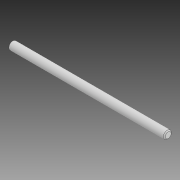
# Autodesk Inventor part: M8x160mm Threaded Rod
Saved by Autodesk Inventor 2020 (Build 240168000, 168)
## iProperties
Created: 2021-06-13
Part Number: M8x160mm Threaded Rod
Material: Generic
Document SubType Name: Modeling
Designer: DDeGo
Density: 1 g/cm^3
Appearance: Default
Author: DDeGo
Autodesk Inventor part; units mm, degrees
ref_plane "YZ Plane" through (0, 0, 0) normal (1, 0, 0) x (0, 1, 0)
ref_plane "XZ Plane" through (0, 0, 0) normal (0, 1, 0) x (-1, 0, 0)
ref_plane "XY Plane" through (0, 0, 0) normal (0, 0, 1) x (1, 0, 0)
sketch "Sketch1" plane through (0, 0, 0) normal (0, 0, 1) x (1, 0, 0)
  line L0 (0, 0) -> (0, 3)
  line L1 (0, 3) -> (-1, 4)
  line L2 (-1, 4) -> (-159, 4)
  line L3 (-159, 4) -> (-160, 3)
  line L4 (-160, 3) -> (-160, 0)
  line L5 (-160, 0) -> (0, 0)
  dimension "d0" = 4
  dimension "d1" = 135
  dimension "d2" = 1
  dimension "d3" = 160
  constraints: 12 end point, 4 perpendicular, 1 parallel, 1 vertical
  measures "d0" distance between parallel lines of L5 L2
  measures "d1" angle of L2 L1
  measures "d2" distance from line of L0.end L2
  measures "d3" distance between parallel lines of L0 L4
revolve "Revolution1" add sketch "Sketch1" angle 360 about axis through (-160, 0, 0) along (1, 0, 0)
body "Solid1"
